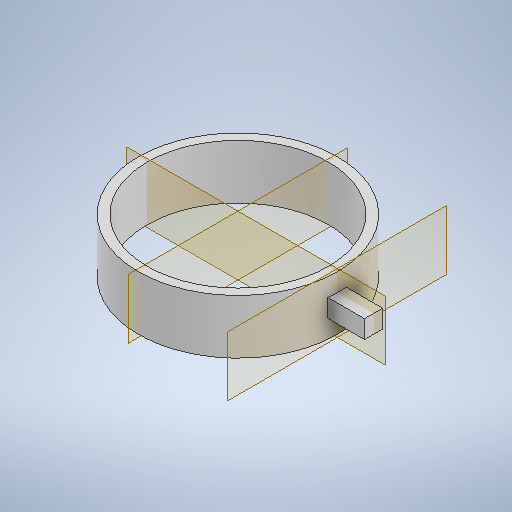
# Autodesk Inventor part: rim
Saved by Autodesk Inventor 2026.1 (Build 301233020, 233B)
## iProperties
Created: 2026-01-04
Part Number: rim
Material: Generic
Document SubType Name: Modeling
Designer: aa992
Density: 1 g/cm^3
Appearance: Default
Author: aa992
Autodesk Inventor part; units mm, degrees
ref_plane "XZ Plane" through (0, 0, 0) normal (0, 1, 0) x (-1, 0, 0)
sketch "Sketch1" plane through (0, 0, 0) normal (0, 1, 0) x (-1, 0, 0)
  circle A0 centre (0, 0) radius 55
  circle A1 centre (0, 0) radius 50
  dimension "d0" = 110
  dimension "d1" = 100
  constraints: 2 centre point, 2 coincident
  measures "d0" diameter of A0
  measures "d1" diameter of A1
extrude "Extrusion1" add sketch "Sketch1" along normal blind 30
ref_plane "Work Plane1" through (55, 0, 0) normal (1, 0, 0) x (0, 1, 0)
sketch "Sketch2" plane through (55, 0, 0) normal (1, 0, 0) x (0, 1, 0)
  line L0 (20, 5) -> (10, 5)
  line L1 (10, 5) -> (10, -5)
  line L2 (10, -5) -> (20, -5)
  line L3 (20, -5) -> (20, 5)
  line L4 (30, -55) -> (30, 55) projected
  line L5 (-6, 0) -> (36, 0) projected
  point P0 (0, 0)
  dimension "d5" = 10
  dimension "d6" = 10
  dimension "d7" = 10
  dimension "d8" = 5
  constraints: 8 end point, 2 parallel, 1 horizontal, 1 perpendicular
  measures "d5" distance of L2.end L0.start
  measures "d6" distance of L1.end L2.end
  measures "d7" distance between parallel lines of L4 L3
  measures "d8" distance between parallel lines of L5 L0
extrude "Extrusion2" add sketch "Sketch2" along normal blind 20
extrude "Extrusion3" add sketch "Sketch2" against normal blind 5
body "Solid1"
